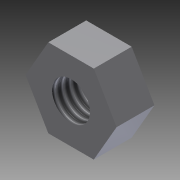
# Autodesk Inventor part: .25 diameter nut
Saved by Autodesk Inventor 2011 SP1 (Build 150282100, 282)
## iProperties
Created: 2013-01-18
Part Number: .25 diameter nut
Document SubType Name: Modeling
Designer: wes
Density: 1 g/cm^3
Author: wes
Autodesk Inventor part; units mm, degrees
ref_plane "YZ Plane" through (0, 0, 0) normal (1, 0, 0) x (0, 1, 0)
ref_plane "XZ Plane" through (0, 0, 0) normal (0, 1, 0) x (-1, 0, 0)
ref_plane "XY Plane" through (0, 0, 0) normal (0, 0, 1) x (1, 0, 0)
sketch "Sketch1" plane through (0, 0, 0) normal (0, 0, 1) x (1, 0, 0)
  line L0 (7.62, 0) -> (3.81, -6.5991)
  line L1 (3.81, -6.5991) -> (-3.81, -6.5991)
  line L2 (-3.81, -6.5991) -> (-7.62, 0)
  line L3 (-7.62, 0) -> (-3.81, 6.5991)
  line L4 (-3.81, 6.5991) -> (3.81, 6.5991)
  line L5 (3.81, 6.5991) -> (7.62, 0)
  circle A0 centre (0, 0) radius 3.175
  dimension "d0" = 6.35
  dimension "d1" = 7.62
  constraints: 12 end point, 2 coincident, 1 centre point, 13 other
  measures "d0" diameter of A0
  measures "d1" distance of point (0, 0) L2.end
extrude "Extrusion1" add sketch "Sketch1" along normal blind 6.35
thread "Thread1" size "1/4-20 UNC" class "2B" standard "ANSI Unified Screw Threads" full length
body "Solid1"
